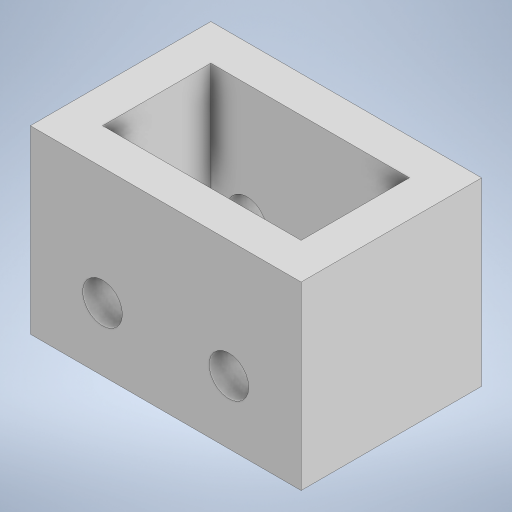
# Autodesk Inventor part: sponge
Saved by Autodesk Inventor 2024.3 (Build 283343000, 343)
## iProperties
Created: 2025-06-10
Part Number: sponge
Material: 一般
Document SubType Name: Modeling
Designer: hikou
Density: 1 g/cm^3
Appearance: 既定
Author: hikou
Autodesk Inventor part; units mm, degrees
ref_plane "YZ Plane" through (0, 0, 0) normal (1, 0, 0) x (0, 1, 0)
ref_plane "XZ Plane" through (0, 0, 0) normal (0, 1, 0) x (-1, 0, 0)
ref_plane "XY Plane" through (0, 0, 0) normal (0, 0, 1) x (1, 0, 0)
sketch "スケッチ1" plane through (0, 0, 0) normal (0, 0, 1) x (1, 0, 0)
  line L0 (-7.5, -5) -> (7.5, -5)
  line L1 (7.5, -5) -> (7.5, 5)
  line L2 (7.5, 5) -> (-7.5, 5)
  line L3 (-7.5, 5) -> (-7.5, -5)
  line L4 (-7.5, -5) -> (7.5, 5) construction
  line L5 (7.5, -5) -> (-7.5, 5) construction
  point P0 (0, 0)
  dimension "d0" = 15
  dimension "d1" = 10
  constraints: 12 end point, 2 midpoint, 2 parallel, 1 horizontal, 1 perpendicular
  measures "d0" distance of L1.end L2.end
  measures "d1" distance of L0.end L1.end
extrude "押し出し1" add sketch "スケッチ1" along normal mid plane 10
sketch "スケッチ2" plane through (-7.5, 5, 5) normal (0, 1, 0) x (1, 0, 0)
  line L0 (13, 2) -> (2, 2)
  line L1 (2, 2) -> (2, 8)
  line L2 (2, 8) -> (13, 8)
  line L3 (13, 8) -> (13, 2)
  line L4 (13, 2) -> (2, 8) construction
  line L5 (2, 2) -> (13, 8) construction
  point P0 (7.5, 5)
  dimension "d4" = 6
  dimension "d5" = 11
  constraints: 12 end point, 2 midpoint, 2 parallel, 1 horizontal, 1 perpendicular
  measures "d4" distance of L0.end L1.end
  measures "d5" distance of L1.end L2.end
extrude "押し出し2" cut sketch "スケッチ2" against normal blind 10
sketch "スケッチ3" plane through (0, 0, -5) normal (0, 0, -1) x (-1, 0, 0)
  line L0 (-7.5, -5) -> (7.5, -5) projected
  line L1 (-7.5, 5) -> (-7.5, -5) projected
  line L2 (7.5, -5) -> (7.5, 5) projected
  point P0 (0, 0)
  point P1 (-3.5, -1.5)
  point P2 (3.5, -1.5)
  dimension "d8" = 3.5
  dimension "d9" = 4
  dimension "d10" = 4
  dimension "d11" = 3.5
  measures "d8" distance from line of L0 point (-3.5, -1.5)
  measures "d9" distance from line of L1 point (-3.5, -1.5)
  measures "d10" distance from line of L2 point (3.5, -1.5)
  measures "d11" distance from line of L0 point (3.5, -1.5)
hole "穴1" at (3.5, -1.5, -5) at (-3.5, -1.5, -5) direction (0, 0, 1) diameter 2.2 end through all
equation "\"d10\" = d9"
equation "\"d11\" = d8"
